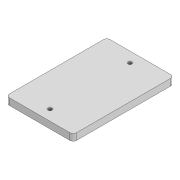
# Autodesk Inventor part: Base
Saved by Autodesk Inventor 2020 (Build 240168000, 168)
## iProperties
Created: 2022-03-14
Part Number: Base
Material: Generic
Document SubType Name: Modeling
Designer: ferrerx
Density: 1 g/cm^3
Appearance: Default
Author: ferrerx
Autodesk Inventor part; units mm, degrees
ref_plane "YZ Plane" through (0, 0, 0) normal (1, 0, 0) x (0, 1, 0)
ref_plane "XZ Plane" through (0, 0, 0) normal (0, 1, 0) x (-1, 0, 0)
ref_plane "XY Plane" through (0, 0, 0) normal (0, 0, 1) x (1, 0, 0)
sketch "Sketch1" plane through (0, 0, 0) normal (0, 1, 0) x (-1, 0, 0)
  line L0 (50, 75) -> (-50, 75)
  line L1 (-50, 75) -> (-50, -75)
  line L2 (-50, -75) -> (50, -75)
  line L3 (50, -75) -> (50, 75)
  line L4 (50, 75) -> (-50, -75) construction
  line L5 (-50, 75) -> (50, -75) construction
  circle A0 centre (0, 59.5) radius 2.8
  line L6 (0, 0) -> (50, 0) construction
  circle A1 centre (0, -59.5) radius 2.8
  dimension "d0" = 150
  dimension "d1" = 100
  dimension "d2" = 59.5
  dimension "d3" = 5.6
  constraints: 14 end point, 3 midpoint, 2 centre point, 2 parallel, 1 horizontal, 1 perpendicular, 1 symmetric about line, 1 other
  measures "d0" distance of L2.end L0.start
  measures "d1" distance of L1.end L2.end
  measures "d2" distance of L6.start A0.centre
  measures "d3" diameter of A0
extrude "Extrusion1" add sketch "Sketch1" along normal blind 10
fillet "Fillet1" radius 5 4 edges at (50, 5, 75) (50, 5, -75) (-50, 5, 75) (-50, 5, -75)
body "Solid1"
